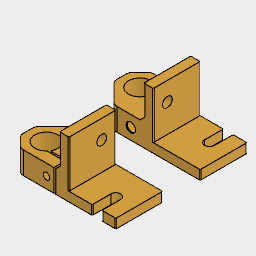
Z_Axis_Linear_Rail_Bracket_1.0_F01 (Autodesk Fusion 360 design; units mm, degrees)
Autodesk Fusion 360 part; units mm, degrees
sketch "スケッチ1" plane through (0, 0, 0) normal (0, 0, 1) x (1, 0, 0)
  circle A0 centre (0, 0) radius 6.2
  line L0 (-10, 10) -> (47, 10)
  line L1 (47, 10) -> (47, -15)
  line L2 (47, -15) -> (-10, -15)
  line L3 (-10, -15) -> (-10, 10)
  line L4 (-10, 10) -> (47, -15) construction
  line L5 (47, 10) -> (-10, -15) construction
  line L6 (22, 10) -> (22, -15)
  line L7 (17, 10) -> (17, -15)
  circle A1 centre (37, 0) radius 2.6
  line L8 (39.6, 10) -> (39.6, 0)
  line L9 (34.4, 10) -> (34.4, 0)
  line L10 (15, 10) -> (15, 3.25)
  line L11 (14, 10) -> (14, 4.25)
  line L12 (14, 4.25) -> (4.5141, 4.25)
  line L13 (15, 3.25) -> (5.2799, 3.25)
  point P0 (18.5, -2.5)
  dimension "d1" = 12.4
  dimension "d2" = 10
  dimension "d3" = 15
  dimension "d4" = 10
  dimension "d5" = 47
  dimension "d6" = 5
  dimension "d7" = 25
  dimension "d8" = 5.2
  dimension "d9" = 10
  dimension "d10" = 15
  dimension "d11" = 2
  dimension "d12" = 1
  dimension "d13" = 5.75
  dimension "d14" = 1
  measures "d1" diameter of A0
  measures "d2" distance of A0.centre L0
  measures "d3" distance of A0.centre L2
  measures "d4" distance of A0.centre L3
  measures "d5" distance of A0.centre L1
  measures "d6" distance of L6 L7
  measures "d7" distance of L1 L6
  measures "d8" diameter of A1
  measures "d9" distance of L1 A1.centre
  measures "d10" distance of L2 A1.centre
  measures "d11" distance of L7 L10
  measures "d12" distance of L10 L11
  measures "d13" distance of L0 L12
  measures "d14" distance of L12 L13
extrude "押し出し1" add sketch "スケッチ1" along normal blind 5 contours L0 L1 L2 L6 A1 L8 L9 makes body 1
extrude "押し出し2" add sketch "スケッチ1" along normal blind 30 contours L0 L2 L6 L7 bodies 1
extrude "押し出し3" add sketch "スケッチ1" along normal blind 12 contours A0 L0 L2 L3 L7 L10 L11 L12 L13 bodies 1
chamfer "面取り1" distance 11 angle 45 1 edges at (-10, -15, 6) on bodies 1
chamfer "面取り2" distance 6 angle 45 1 edges at (-10, 10, 6) on bodies 1
chamfer "面取り3" distance 2 angle 45 1 edges at (17, -2.5, 12) on bodies 1
fillet "フィレット1" radius 0.5 10 edges at (47, 10, 2.5) (39.6, 10, 2.5) (34.4, 10, 2.5) (22, 10, 17.5) (17, 10, 22) (5.2799, 3.25, 6) (4.5141, 4.25, 6) (17, -15, 22) (22, -15, 17.5) (47, -15, 2.5) on bodies 1
fillet "フィレット2" radius 4 4 edges at (-4, 10, 6) (-10, 4, 6) (-10, -4, 6) (1, -15, 6) on bodies 1
hole "穴1" at (17, -7.5, 20) direction (1, 0, 0) diameter 5.2 depth 10 tip angle 118 bodies 1
hole "穴2" at (10, 10, 6) direction (0, -1, 0) diameter 3.5 depth 30 tip angle 118 bodies 1
sketch "スケッチ2" plane through (0, -15, 0) normal (0, -1, 0) x (1, 0, 0)
  circle A0 centre (10, 6) radius 1.75
  line L0 (2.6569, 12) -> (2.6569, 0)
  line L1 (2.6569, 0) -> (46.5, 0)
  line L2 (46.5, 0) -> (46.5, 5)
  line L3 (46.5, 5) -> (21.5, 5)
  line L4 (21.5, 5) -> (21.5, 30)
  line L5 (21.5, 30) -> (17.5, 30)
  line L6 (17.5, 30) -> (17.5, 14.5)
  line L7 (17.5, 14.5) -> (15, 12)
  line L8 (15, 12) -> (2.6569, 12)
  circle A1 centre (10, 6) radius 2.5
  circle A2 centre (10, 6) radius 2.35
  dimension "d36" = 5
  dimension "d37" = 4.7
  measures "d36" diameter of A1
  measures "d37" diameter of A2
extrude "押し出し4" cut sketch "スケッチ2" against normal blind 5 contours A2 bodies 1
extrude "押し出し5" cut sketch "スケッチ2" against normal blind 0.5 contours A1 bodies 1
ref_plane "作業平面1" through (0, -25, 0) normal (0, 1, 0) x (0, 0, 1)
mirror "ミラー1" about plane through (0, -25, 0) normal (0, 1, 0) of bodies 1 makes body 2
